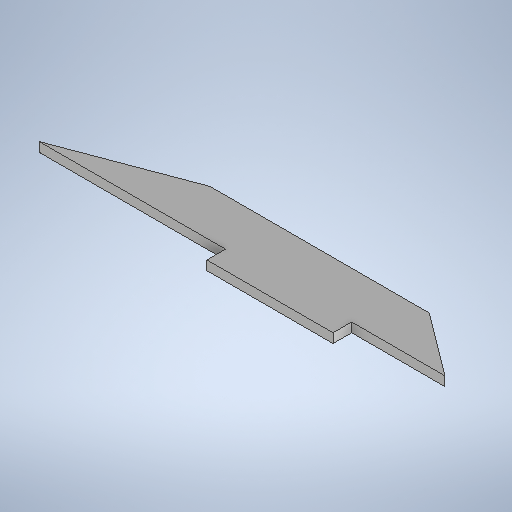
# Autodesk Inventor part: Moving Ramp Inside Rail
Saved by Autodesk Inventor 2025.1 (Build 291241020, 241B)
## iProperties
Created: 2024-10-27
Part Number: Moving Ramp Inside Rail
Material: Generic
Document SubType Name: Modeling
Designer: aly_g
Density: 1 g/cm^3
Appearance: Default
Mass: 4.1328 g
Surface Area: 34.4796 cm^2
Volume: 4.1328 cm^3
Author: aly_g
Autodesk Inventor part; units mm, degrees
ref_plane "YZ Plane" through (0, 0, 0) normal (1, 0, 0) x (0, 1, 0)
ref_plane "XZ Plane" through (0, 0, 0) normal (0, 1, 0) x (-1, 0, 0)
ref_plane "XY Plane" through (0, 0, 0) normal (0, 0, 1) x (1, 0, 0)
sketch "Sketch1" plane through (0, 0, 0) normal (0, 0, 1) x (1, 0, 0)
  line L0 (60, -6) -> (60, 0)
  line L1 (100.6, 0) -> (115.6, 0)
  line L2 (0, 0) -> (60, 0)
  line L3 (100.6, 0) -> (130.6, 0)
  line L4 (60, -6) -> (100.6, -6)
  line L5 (100.6, -6) -> (100.6, 0)
  line L6 (0, 0) -> (40, 15)
  line L7 (40, 15) -> (110.6, 15)
  line L8 (110.6, 15) -> (130.6, 0)
  dimension "d24" = 6
  dimension "d26" = 60
  dimension "d27" = 40.6
  dimension "d28" = 30
  dimension "d29" = 15
  dimension "d30" = 40
  dimension "d31" = 20
  constraints: 18 end point, 5 horizontal, 2 perpendicular, 1 midpoint, 1 parallel
  measures "d24" distance of L4.end L1.start
  measures "d26" distance of L2.start L0.end
  measures "d27" distance of L0.start L4.end
  measures "d28" distance of L1.start L3.end
  measures "d29" vertical distance of L7.end L3.end
  measures "d30" horizontal distance of L2.start L6.end
  measures "d31" horizontal distance of L7.end L3.end
extrude "Extrusion1" add sketch "Sketch1" along normal blind 3
body "Solid1"
